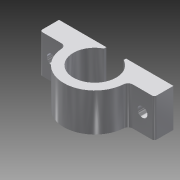
# Autodesk Inventor part: Bearing Block V1.500 Drivetrain
Saved by Autodesk Inventor 2013 (Build 170138000, 138)
## iProperties
Created: 2013-01-06
Part Number: Bearing Block V1.500 Drivetrain
Material: Aluminum 6061
Document SubType Name: Modeling
Designer: Moses
Density: 2.71 g/cm^3
Mass: 70.2087 g
Surface Area: 93.0726 cm^2
Volume: 25.9073 cm^3
Author: Moses
Autodesk Inventor part; units mm, degrees
ref_plane "YZ Plane" through (0, 0, 0) normal (1, 0, 0) x (0, 1, 0)
ref_plane "XZ Plane" through (0, 0, 0) normal (0, 1, 0) x (-1, 0, 0)
ref_plane "XY Plane" through (0, 0, 0) normal (0, 0, 1) x (1, 0, 0)
sketch "Sketch1" plane through (0, 0, 0) normal (0, 1, 0) x (-1, 0, 0)
  line L0 (0, 0) -> (38.1, 0)
  line L1 (38.1, 0) -> (38.1, 34.925)
  line L2 (38.1, 34.925) -> (0, 34.925)
  line L3 (0, 34.925) -> (0, 0)
  line L4 (19.05, 34.925) -> (19.05, 0) construction
  line L5 (-19.05, 12.7) -> (-19.05, 0)
  line L6 (-19.05, 0) -> (0, 0)
  line L7 (57.15, 12.7) -> (57.15, 0)
  line L8 (57.15, 0) -> (38.1, 0)
  line L9 (-19.05, 12.7) -> (0, 12.7)
  line L10 (38.1, 12.7) -> (57.15, 12.7)
  line L11 (0, 14.2875) -> (38.1, 14.2875) construction
  circle A0 centre (19.05, 14.2875) radius 14.2875
  line L12 (12.5046, 1.5875) -> (12.5046, 0)
  line L13 (25.5954, 1.5875) -> (25.5954, 0)
  arc A1 (39.6264, 12.7) -> (-1.5264, 12.7) centre (19.05, 14.2875) ccw
  point P0 (0, 22.225)
  point P1 (38.1, 22.225)
  dimension "d0" = 38.1
  dimension "d1" = 34.925
  dimension "d9" = 12.7
  dimension "d10" = 19.05
  dimension "d11" = 19.05
  dimension "d12" = 12.7
  dimension "d21" = 28.575
  dimension "d22" = 14.2875
  dimension "d34" = 1.5875
  constraints: 28 end point, 10 point on line, 7 parallel, 6 point on circle, 3 midpoint, 3 perpendicular, 2 centre point, 2 horizontal, 1 coincident, 1 collinear, 1 tangent, 1 vertical
  measures "d0" distance of L2.end L1.end
  measures "d1" distance of L1.end L0.end
  measures "d9" distance of L5.start L5.end
  measures "d10" distance of L5.end L0.start
  measures "d11" distance of L7.end L0.end
  measures "d12" distance of L7.start L7.end
  measures "d21" diameter of A0
  measures "d22" distance between parallel lines of L0 L11
  measures "d34" distance of L12.start L12.end
extrude "Extrusion1" add sketch "Sketch1" along normal blind 25.4 contours L3 A1 L1 L0 L13 A0 L12 | L6 L5 L9 L3 | L9 A1 L3 | L1 L10 L7 L8 | A1 L10 L1
fillet "Fillet1" radius 3.175 2 edges at (-39.6264, 12.7, 12.7) (1.5264, 12.7, 12.7)
fillet "Fillet1" radius 1.5875 2 edges at (19.05, 12.7, 12.7) (-57.15, 12.7, 12.7)
sketch "Sketch2" plane through (19.05, 25.4, 0) normal (0, 0, -1) x (-1, 0, 0)
  line L0 (14.3405, 0) -> (1.5875, 0) construction
  line L1 (74.6125, 0) -> (61.8595, 0) construction
  circle A0 centre (7.9375, -12.7) radius 3.302
  circle A1 centre (68.2625, -12.7) radius 3.302
  line L2 (74.6125, -25.4) -> (61.8595, -25.4) projected
  line L3 (14.3405, -25.4) -> (1.5875, -25.4) projected
  line L4 (74.6125, -25.4) -> (74.6125, 0) construction
  line L5 (1.5875, 0) -> (1.5875, -25.4) construction
  line L6 (0, -12.7) -> (76.2, -12.7) construction
  line L7 (38.1, 0) -> (38.1, -25.4) construction
  line L8 (23.8125, 0) -> (52.3875, 0) projected
  line L9 (23.8125, -25.4) -> (52.3875, -25.4) projected
  line L10 (0, -25.4) -> (0, 0) projected
  line L11 (76.2, -25.4) -> (76.2, 0) projected
  line L12 (61.8595, 0) -> (61.8595, -25.4) projected
  line L13 (14.3405, -25.4) -> (14.3405, 0) projected
  point P0 (31.5546, 0)
  point P1 (31.5546, -25.4)
  point P2 (38.1, 0)
  dimension "d15" = 6.604
  dimension "d16" = 6.604
  dimension "d24" = 30.1625
  dimension "d25" = 30.1625
  dimension "d26" = 60.325
  constraints: 4 end point, 4 midpoint, 4 point on line, 2 centre point
  measures "d15" diameter of A0
  measures "d16" diameter of A1
  measures "d24" distance from line of A1.centre L7
  measures "d25" distance from line of A0.centre L7
  measures "d26" distance of A1.centre A0.centre
extrude "Extrusion3" cut sketch "Sketch2" against normal through all
equation "\"d9\" = d12"
equation "\"d11\" = d10"
equation "\"d15\" = d16"
equation "\"d25\" = d24"
body "Solid1"
